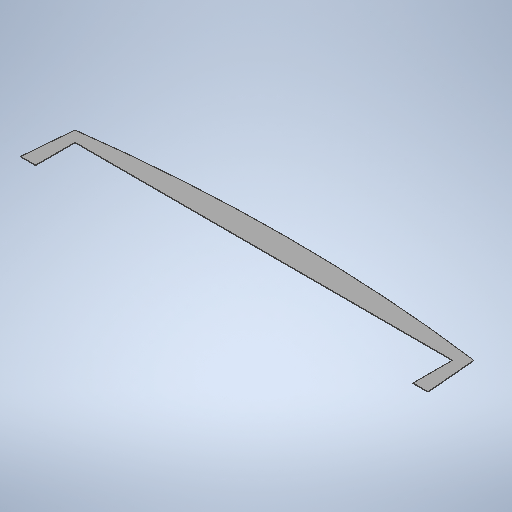
# Autodesk Inventor part: MSC 0511 rib back mould
Saved by Autodesk Inventor 2025 (Build 290162010, 162A)
## iProperties
Created: 2024-04-28
Part Number: MSC 0511 rib back mould
Material: Stainless Steel
Document SubType Name: Sheet Metal
Designer: admin
Stock Number: МОО 051 шпангоут спина
Density: 8 g/cm^3
Flat Pattern Width: 23.8564 cm
Flat Pattern Length: 153.274 cm
Flat Pattern Area: 3656.57 cm^2
Sheet Metal Rule: AISI304 2mm Die16
Sheet Metal Width: 238,564 mm
Sheet Metal Length: 1532,742 mm
Sheet Metal Area: 365657,070 mm^2
Appearance: Default
Author: admin
Стрингер_2: 67,669 mm
Стрингер_1: 51,765 mm
Autodesk Inventor part; units mm, degrees
ref_plane "YZ Plane" through (0, 0, 0) normal (1, 0, 0) x (0, 1, 0)
ref_plane "XZ Plane" through (0, 0, 0) normal (0, 1, 0) x (-1, 0, 0)
ref_plane "XY Plane" through (0, 0, 0) normal (0, 0, 1) x (1, 0, 0)
sketch "Sketch1" plane through (0, 0, 0) normal (0, 0, 1) x (1, 0, 0)
  line L0 (-750, 0) -> (750, 0) construction
  line L1 (750, 0) -> (750, -2700) construction
  line L2 (750, -2700) -> (-750, -2700) construction
  line L3 (-750, -2700) -> (-750, 0) construction
  line L4 (800, 50) -> (-800, 50)
  line L5 (-800, 50) -> (-800, -2750) construction
  line L6 (-800, -2750) -> (800, -2750) construction
  line L7 (800, -2750) -> (800, 50) construction
  line L8 (-850, 100) -> (850, 100)
  line L9 (850, 100) -> (850, -2800) construction
  line L10 (850, -2800) -> (-850, -2800) construction
  line L11 (-850, -2800) -> (-850, 100) construction
  arc A0 (750, 0) -> (746.2569, 0.5) centre (0, -5600) ccw construction
  line L12 (-750, -2100) -> (750, -2100) construction
  line L13 (114.1118, -2698.3696) -> (750, -2100) construction
  arc A1 (750, -2100) -> (770.156, -238.4205) centre (-10250, -1050) ccw construction
  line L14 (750, 0) -> (749.6018, -2.9735) construction
  arc A2 (750, -3.0268) -> (0, 47) centre (-0.2, -5603) ccw construction
  line L15 (750, 0) -> (747.0136, -0.2851) construction
  arc A3 (767.1641, -238.6409) -> (747.4657, -5.0326) centre (-10252.9895, -1050.2527) ccw construction
  arc A4 (750.3581, -3.7586) -> (746.2569, 0.5) centre (745.6295, -4.2083) ccw
  arc A5 (747.4657, -5.0326) -> (744.8748, -2.3426) centre (744.4792, -5.3164) ccw construction
  line L16 (750, -2100) -> (752.9864, -2100.2851) construction
  arc A6 (752.9864, -2100.2851) -> (771.2831, -213.263) centre (-10246.9891, -1050.0292) ccw
  line L17 (750, -2100) -> (752.0559, -2102.1848) construction
  arc A7 (749.1768, -2100.7746) -> (750.1074, -2098.8746) centre (747.1209, -2098.5898) ccw construction
  line L18 (0, -2697) -> (110, -2697) construction
  line L19 (112.0559, -2696.1848) -> (685.3133, -2156.7506) construction
  arc A8 (110, -2700) -> (114.1118, -2698.3696) centre (110, -2694) ccw construction
  arc A9 (110, -2697) -> (112.0559, -2696.1848) centre (110, -2694) ccw construction
  line L20 (685.3133, -2156.7506) -> (687.3692, -2158.9354) construction
  line L21 (752.0559, -2102.1848) -> (671.2185, -2178.2526) construction
  line L22 (671.2185, -2178.2526) -> (669.1626, -2176.0678) construction
  arc A10 (747.4657, -5.0326) -> (747.0136, -0.2851) centre (-10252.9895, -1050.2527) ccw construction
  arc A11 (746.2569, 0.5) -> (0, 50) centre (0, -5600) ccw
  arc A12 (750.3581, -3.7586) -> (750, 0) centre (-10250, -1050) ccw construction
  line L23 (770.156, -238.4205) -> (767.1641, -238.6409) construction
  line L24 (768.2917, -213.4901) -> (771.2831, -213.263) construction
  arc A13 (770.156, -238.4205) -> (750.3581, -3.7586) centre (-10250, -1050) ccw
  line L25 (0, 100) -> (0, 50)
  line L26 (0, -2700) -> (0, -2697) construction
  line L27 (0, 47) -> (0, 0) construction
  line L28 (0, 50) -> (0, 47)
  arc A14 (752.0559, -2102.1848) -> (752.9864, -2100.2851) centre (749.9998, -2099.9999) ccw construction
  circle A15 centre (768.2917, -213.4901) radius 25
  line L29 (850, -258.4205) -> (774.6194, -258.4205) construction
  arc A16 (800, 50) -> (0, 100) centre (0, -6325) ccw construction
  arc A17 (824.6194, -258.4205) -> (800, 50) centre (-10711.2413, -1024.069) ccw construction
  line L30 (824.6194, -258.4205) -> (824.6194, 100) construction
  line L31 (-25, 100) -> (-25, 50) construction
  line L32 (778.0966, -308.4205) -> (850, -308.4205) construction
  line L33 (0, -308.4205) -> (0, 47)
  line L34 (0, -40) -> (753.7448, -40)
  line L35 (710, -40) -> (710, -188.564)
  line L36 (710, -188.564) -> (766.3709, -188.564)
  point P0 (0, 0)
  point P1 (0, 0)
  point P2 (0, -2750)
  point P3 (766.3709, -188.564)
  point P4 (773.135, -238.0165)
  dimension "d6" = 1500
  dimension "d7" = 2700
  dimension "d8" = 2100
  dimension "d9" = 4.75
  dimension "d10" = 3
  dimension "d11" = 3
  dimension "d12" = 6
  dimension "d13" = 3
  dimension "d14" = 239.271
  dimension "d15" = 50
  dimension "d16" = 50
  dimension "d17" = 3
  dimension "d18" = 110
  dimension "d19" = 25
  dimension "d20" = 111
  dimension "d21" = 25
  dimension "d34" = 20
  dimension "d35" = 50
  dimension "d47" = 25
  dimension "d49" = 50
  dimension "d91" = 40
  dimension "d92" = 40
  measures "d6" distance of L3.end L1.start
  measures "d7" distance of L1.start L1.end
  measures "d8" distance between parallel lines of L12 L0
  measures "d9" radius of A4
  measures "d10" radius of A5
  measures "d11" radius of A7
  measures "d12" radius of A8
  measures "d13" radius of A9
  measures "d14" distance of L23.start L1.start
  measures "d15" distance between parallel lines of L4 L8
  measures "d16" distance between parallel lines of L0 L4
  measures "d17" distance of L28.start L27.start
  measures "d18" distance from line of L26 A8.centre
  measures "d19" distance of L22.end L20.end
  measures "d20" distance of L16.start L22.end
  measures "d21" distance of L23.start L24.start
  measures "d34" vertical distance of L23.start L29.end
  measures "d35" distance of L30.start L29.end
  measures "d47" distance between parallel lines of L25 L31
  measures "d49" distance of L32.end L29.start
  measures "d91" distance between parallel lines of L34 L0
  measures "d92" distance between parallel lines of L35 L1
extrude "Plate3" add sketch "Sketch1" along normal blind 2 contours A13 L34 L33 L28 A11 A4 | A13 L36 L35 L34
mirror "Mirror1" about plane through (0, 0, 0) normal (1, 0, 0)
equation "\"d6\" = d22"
equation "\"d7\" = d23"
equation "\"d8\" = d24"
equation "\"d10\" = d26"
equation "\"d11\" = d27"
equation "\"d12\" = d27 + d31"
equation "\"d13\" = d27"
equation "\"d14\" = d28"
equation "\"d17\" = d27"
equation "\"d18\" = 0.5 * d32"
equation "\"d19\" = d29"
equation "\"d20\" = Бак_борт_длина_фланца"
equation "\"d21\" = d29"
equation "\"d35\" = d15"
equation "\"d47\" = Усилитель_нахлест"
equation "\"d49\" = 2 * Усилитель_нахлест"
equation "\"BendReliefWidth\" = Thickness"
equation "\"BendReliefDepth\" = 0.5 * Thickness"
equation "\"CornerReliefSize\" = 4 * Thickness"
equation "\"MinimumRemnant\" = 2 * Thickness"
equation "\"GapSize\" = Thickness"
equation "\"d25\" = d27 + d31"
equation "\"d26\" = d27"
equation "\"d31\" = d27"
equation "\"Стрингер_2\" = 67.66905"
equation "\"Стрингер_1\" = 51.76503"
equation "\"d22\" = 1500"
equation "\"d23\" = 2700"
equation "\"d24\" = 2100"
equation "\"d27\" = 3"
equation "\"d28\" = 239.271"
equation "\"d32\" = 220"
equation "\"d29\" = 25"
equation "\"Бак_борт_длина_фланца\" = 111"
equation "\"Усилитель_нахлест\" = 25"
equation "\"Thickness\" = 2"
body "Solid2"
